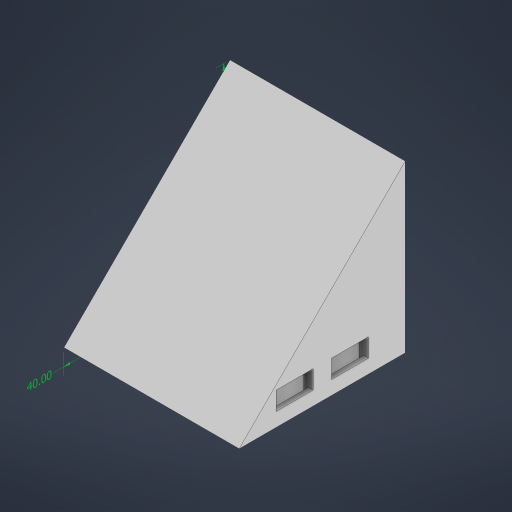
# Autodesk Inventor part: ramp
Saved by Autodesk Inventor 2024 (Build 280153000, 153)
## iProperties
Created: 2023-06-19
Part Number: ramp
Material: 일반
Document SubType Name: Modeling
Designer: 6gioc
Density: 1 g/cm^3
Appearance: 기본값
Author: 6gioc
Autodesk Inventor part; units mm, degrees
ref_plane "YZ Plane" through (0, 0, 0) normal (1, 0, 0) x (0, 1, 0)
ref_plane "XZ Plane" through (0, 0, 0) normal (0, 1, 0) x (-1, 0, 0)
ref_plane "XY Plane" through (0, 0, 0) normal (0, 0, 1) x (1, 0, 0)
sketch "스케치1" plane through (0, 0, 0) normal (1, 0, 0) x (0, 1, 0)
  line L0 (0, 0) -> (180, 0)
  line L1 (180, 0) -> (180, -180)
  line L2 (180, -180) -> (0, -180)
  line L3 (0, -180) -> (0, 0)
  line L4 (0, 0) -> (180, -180)
  dimension "d0" = 180
  dimension "d1" = 180
  constraints: 10 end point, 2 parallel, 1 horizontal, 1 perpendicular
  measures "d0" distance of L1.end L2.end
  measures "d1" distance of L0.end L1.end
extrude "돌출1" add sketch "스케치1" along normal blind 190 contours L4 L2 L3
sketch "스케치2" plane through (0, 0, 0) normal (-1, 0, 0) x (0, 0, 1)
  line L0 (-140, 15) -> (-100, 15)
  line L1 (-100, 15) -> (-100, 35)
  line L2 (-100, 35) -> (-140, 35)
  line L3 (-140, 35) -> (-140, 15)
  line L4 (-80, 35) -> (-40, 35)
  line L5 (-40, 35) -> (-40, 15)
  line L6 (-40, 15) -> (-80, 15)
  line L7 (-80, 15) -> (-80, 35)
  line L8 (-180, 0) -> (-180, 180) projected
  line L9 (0, 0) -> (-180, 0) projected
  point P0 (-140, 25)
  point P1 (-80, 25)
  dimension "d4" = 40
  dimension "d5" = 20
  dimension "d6" = 40
  dimension "d7" = 20
  dimension "d8" = 40
  dimension "d9" = 20
  dimension "d10" = 15
  dimension "d11" = 15
  dimension "d46" = 40
  constraints: 16 end point, 4 parallel, 2 horizontal, 2 midpoint, 2 perpendicular, 1 point on line
  measures "d4" distance of L2.end L1.end
  measures "d5" distance of L1.end L0.end
  measures "d6" distance of L5.end L6.end
  measures "d7" distance of L4.end L5.end
  measures "d8" distance from line of L8 point (-140, 25)
  measures "d9" distance from line of point (-80, 25) L1
  measures "d10" distance between parallel lines of L9 L0
  measures "d11" distance between parallel lines of L9 L6
  measures "d46" distance from line of L9.start L5
extrude "돌출2" cut sketch "스케치2" against normal blind 10
sketch "스케치3" plane through (0, 15, -40) normal (0, 1, 0) x (1, 0, 0)
  line L0 (10, 0) -> (10, 40) projected
  line L1 (10, 0) -> (5, 0)
  line L2 (5, 0) -> (5, 40)
  line L3 (5, 40) -> (10, 40)
  line L4 (10, 40) -> (10, 0)
  line L5 (10, 100) -> (5, 100)
  line L6 (5, 100) -> (5, 60)
  line L7 (5, 60) -> (10, 60)
  line L8 (10, 60) -> (10, 100)
  point P0 (0, -40)
  dimension "d14" = 5
  dimension "d15" = 40
  dimension "d16" = 5
  dimension "d17" = 40
  constraints: 16 end point, 4 parallel, 2 horizontal, 2 perpendicular
  measures "d14" distance of L2.end L3.end
  measures "d15" distance of L1.end L2.end
  measures "d16" distance of L7.end L6.end
  measures "d17" distance of L6.end L5.end
extrude "돌출3" cut sketch "스케치3" against normal blind 10
sketch "스케치4" plane through (190, 0, 0) normal (1, 0, 0) x (0, 0, -1)
  line L0 (140, 35) -> (100, 35)
  line L1 (100, 35) -> (100, 15)
  line L2 (100, 15) -> (140, 15)
  line L3 (140, 15) -> (140, 35)
  line L4 (80, 35) -> (40, 35)
  line L5 (40, 35) -> (40, 15)
  line L6 (40, 15) -> (80, 15)
  line L7 (80, 15) -> (80, 35)
  line L8 (180, 0) -> (180, 180) projected
  line L9 (0, 0) -> (180, 0) projected
  point P0 (140, 25)
  dimension "d20" = 40
  dimension "d21" = 20
  dimension "d22" = 40
  dimension "d23" = 20
  dimension "d24" = 20
  dimension "d25" = 40
  dimension "d26" = 15
  constraints: 16 end point, 4 parallel, 2 horizontal, 2 perpendicular, 1 midpoint, 1 point on line
  measures "d20" distance of L2.end L1.end
  measures "d21" distance of L1.end L0.end
  measures "d22" distance of L6.end L5.end
  measures "d23" distance of L5.end L4.end
  measures "d24" distance between parallel lines of L1 L7
  measures "d25" distance from line of L8 point (140, 25)
  measures "d26" distance between parallel lines of L9 L2
extrude "돌출4" cut sketch "스케치4" against normal blind 10
sketch "스케치5" plane through (190, 15, -40) normal (0, 1, 0) x (1, 0, 0)
  line L0 (0, 0) -> (-10, 0) projected
  line L1 (-10, 0) -> (-5, 0)
  line L2 (-5, 0) -> (-5, 40)
  line L3 (-5, 40) -> (-10, 40)
  line L4 (-10, 40) -> (-10, 0)
  line L5 (-10, 60) -> (-5, 60)
  line L6 (-5, 60) -> (-5, 100)
  line L7 (-5, 100) -> (-10, 100)
  line L8 (-10, 100) -> (-10, 60)
  point P0 (-190, -40)
  dimension "d29" = 5
  dimension "d30" = 40
  dimension "d31" = 5
  dimension "d32" = 40
  constraints: 16 end point, 4 parallel, 2 horizontal, 2 perpendicular
  measures "d29" distance of L3.end L2.end
  measures "d30" distance of L2.end L1.end
  measures "d31" distance of L7.end L6.end
  measures "d32" distance of L6.end L5.end
extrude "돌출5" cut sketch "스케치5" against normal blind 10
